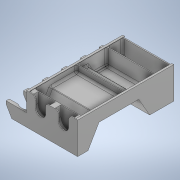
# Autodesk Inventor part: CardboardTray
Saved by Autodesk Inventor 2021 (Build 250183000, 183)
## iProperties
Created: 2023-03-18
Part Number: CardboardTray
Material: ABS Plastic
Document SubType Name: Modeling
Designer: Bradley
Density: 1.06 g/cm^3
Appearance: Smooth - Medium Gray
Author: Bradley
Autodesk Inventor part; units mm, degrees
ref_plane "YZ Plane" through (0, 0, 0) normal (1, 0, 0) x (0, 1, 0)
ref_plane "XZ Plane" through (0, 0, 0) normal (0, 1, 0) x (-1, 0, 0)
ref_plane "XY Plane" through (0, 0, 0) normal (0, 0, 1) x (1, 0, 0)
sketch "Sketch1" plane through (0, 0, 0) normal (1, 0, 0) x (0, 1, 0)
  line L0 (-22.4, 71.125) -> (-22.4, 55.7645)
  line L1 (-22.4, 55.7645) -> (5.9, 39.4255)
  line L2 (5.9, 39.4255) -> (5.9, -19.1755)
  line L3 (5.9, -19.1755) -> (-22.4, -35.5145)
  line L4 (-22.4, -35.5145) -> (-22.4, -71.125)
  line L5 (-22.4, -71.125) -> (22.4, -71.125)
  line L6 (22.4, -71.125) -> (22.4, 71.125)
  line L7 (22.4, 71.125) -> (-22.4, 71.125)
  line L8 (5.65, 39.2812) -> (5.65, -19.0312) construction
  line L9 (5.65, -19.0312) -> (-44.85, -48.1874) construction
  line L10 (-44.85, -48.1874) -> (-95.35, -19.0312) construction
  line L11 (-95.35, -19.0312) -> (-95.35, 39.2812) construction
  line L12 (-95.35, 39.2812) -> (-44.85, 68.4374) construction
  line L13 (-44.85, 68.4374) -> (5.65, 39.2812) construction
  line L14 (5.9, 39.4255) -> (5.9, -19.1755) construction
  line L15 (5.9, -19.1755) -> (-44.85, -48.4761) construction
  line L16 (-44.85, -48.4761) -> (-95.6, -19.1755) construction
  line L17 (-95.6, -19.1755) -> (-95.6, 39.4255) construction
  line L18 (-95.6, 39.4255) -> (-44.85, 68.7261) construction
  line L19 (-44.85, 68.7261) -> (5.9, 39.4255) construction
  line L20 (-22.4, -35.5145) -> (-22.4, 55.7645)
  point P0 (5.9, 10.125)
  point P1 (5.9, 10.125)
  point P2 (-44.85, 10.125)
  point P3 (0, 0)
  point P4 (22.4, 0)
  point P5 (0, 71.125)
  dimension "d0" = 101
  dimension "d1" = 61
  dimension "d2" = 0.25
  dimension "d3" = 73.2
  dimension "d4" = 142.25
  dimension "d5" = 44.8
  dimension "d80" = 16.5
  constraints: 42 end point, 3 collinear, 3 midpoint, 3 parallel, 3 perpendicular, 3 vertical, 2 point on line, 1 coincident, 1 horizontal alignment, 1 vertical alignment, 18 other
  measures "d0" distance between parallel lines of L11 L8
  measures "d1" distance from line of point (-44.85, 10.125) L7
  measures "d2" distance between parallel lines of L13 L19
  measures "d3" distance between parallel lines of L0 L17
  measures "d4" distance of L5.end L6.end
  measures "d5" distance of L6.end L0.start
  measures "d80" distance between parallel lines of L6 L2
extrude "Extrusion1" add sketch "Sketch1" along normal blind 64.6 contours L7 L6 L5 L4 L3 L2 L1 L0
extrude "Extrusion2" add sketch "Sketch1" against normal blind 11
sketch "Sketch2" plane through (64.6, -22.4, 71.125) normal (0, 0, 1) x (1, 0, 0)
  line L0 (-75.6, 0) -> (0, 0) projected
  line L1 (0, 44.8) -> (0, 0) projected
  line L2 (-75.6, 44.8) -> (0, 44.8) projected
  line L3 (-75.6, 0) -> (-75.6, 44.8) projected
  line L4 (-87.5152, -18) -> (-118.8076, -72.2) construction
  line L5 (-118.8076, -72.2) -> (-181.3924, -72.2) construction
  line L6 (-181.3924, -72.2) -> (-212.6848, -18) construction
  line L7 (-212.6848, -18) -> (-181.3924, 36.2) construction
  line L8 (-181.3924, 36.2) -> (-118.8076, 36.2) construction
  line L9 (-118.8076, 36.2) -> (-87.5152, -18) construction
  line L10 (-118.5189, 36.7) -> (-181.6811, 36.7) construction
  line L11 (-181.6811, 36.7) -> (-213.2621, -18) construction
  line L12 (-213.2621, -18) -> (-181.6811, -72.7) construction
  line L13 (-181.6811, -72.7) -> (-118.5189, -72.7) construction
  line L14 (-118.5189, -72.7) -> (-86.9379, -18) construction
  line L15 (-86.9379, -18) -> (-118.5189, 36.7) construction
  line L16 (-75.6, 0) -> (-97.3302, 0)
  line L17 (-97.3302, 0) -> (-105.6, 14.3237)
  line L18 (-105.6, 14.3237) -> (-105.6, 18.8)
  line L19 (-105.6, 18.8) -> (-75.6, 18.8)
  point P0 (-64.6, 22.4)
  point P1 (-150.1, -18)
  point P2 (-64.6, -73.2)
  point P3 (-64.6, -73.2)
  point P4 (-64.6, -73.2)
  dimension "d10" = 150.1
  dimension "d11" = 108.4
  dimension "d12" = 0.5
  dimension "d13" = 1
  dimension "d14" = 92
  dimension "d15" = 30
  dimension "d51" = 18.8
  dimension "d52" = 26
  constraints: 32 end point, 3 point on line, 2 horizontal, 1 perpendicular, 1 vertical, 18 other
  measures "d10" distance from line of point (-150.1, -18) L1
  measures "d11" distance between parallel lines of L5 L8
  measures "d12" distance between parallel lines of L8 L10
  measures "d13" distance from line of point (-64.6, -73.2) L5
  measures "d14" distance from line of point (-64.6, -73.2) L19
  measures "d15" distance between parallel lines of L18 L3
  measures "d51" distance between parallel lines of L16 L19
  measures "d52" distance between parallel lines of L2 L19
extrude "Extrusion3" add sketch "Sketch2" against normal up to surface (142.25 mm away) contours L16 L17 L18 L19 L3
sketch "Sketch6" plane through (-41, -3.6, 71.125) normal (0, 1, 0) x (1, 0, 0)
  circle A0 centre (21.0198, 15.0417) radius 12.75 construction
  circle A1 centre (21.0198, 15.0417) radius 13
  line L0 (30, 142.25) -> (0, 142.25) projected
  line L1 (0, 0) -> (0, 142.25) projected
  line L2 (30, 0) -> (0, 0) projected
  line L3 (30, 142.25) -> (30, 0) projected
  circle A2 centre (21.0198, 15.0417) radius 15.0417 construction
  line L4 (8.2698, 0) -> (105.6, 0) construction
  line L5 (8.2698, 0) -> (8.2698, 142.25) projected
  line L6 (0, 0) -> (0, 142.25) projected
  line L7 (0, 4.5417) -> (13.355, 4.5417)
  line L8 (13.355, 4.5417) -> (13.355, 25.5417)
  line L9 (13.355, 25.5417) -> (0, 25.5417)
  line L10 (0, 25.5417) -> (0, 4.5417)
  arc A3 (10.355, 4.5417) -> (10.355, 25.5417) centre (-6.52, 15.0417) ccw
  circle A4 centre (21.0198, 127.2083) radius 15.0417
  line L11 (21.0198, 15.0417) -> (21.0198, 127.2083) construction
  line L12 (30, 142.25) -> (0, 142.25) construction
  circle A5 centre (21.0198, 43.0833) radius 15.0417 construction
  point P0 (41, 71.125)
  point P1 (0, 25.5417)
  point P2 (30, 5.6419)
  point P3 (30, 24.4415)
  dimension "d43" = 25.5
  dimension "d44" = 2.0417
  dimension "d45" = 26
  dimension "d46" = 21
  dimension "d53" = 3
  dimension "d59" = 112.1667
  dimension "d60" = 30.0833
  dimension "d61" = 28.0417
  constraints: 10 end point, 6 centre point, 5 tangent, 4 point on circle, 4 point on line, 2 coincident, 2 equal radius, 2 parallel, 1 horizontal, 1 horizontal alignment, 1 perpendicular, 1 vertical
  measures "d43" diameter of A0
  measures "d44" radial gap between concentric circles of A1 A2
  measures "d45" diameter of A1
  measures "d46" distance of L7.end L8.end
  measures "d53" distance from line of A3.end L8
  measures "d59" distance of L11.start L11.end
  measures "d60" diameter of A2
  measures "d61" distance of A5.centre A0.centre
extrude "Extrusion5" cut sketch "Sketch6" along normal blind 26 and the other way blind 17.8 contours A1 L3 | L3 A1 L8 | L8 A3 A1 | A1 A3 L9 | L7 A3 A1 | A1 A3 L8 | A3 A1 L5 | A1 L5 L9 A3 | A3 L7 L5 A1 | L5 A1 | A1 L5 L7 L1 L9
extrude "Extrusion6" cut sketch "Sketch6" against normal through all contours A3 A1 L5 | A1 L5 L9 A3 | A3 L7 L5 A1 | L5 A1 | A1 L5 L7 L1 L9
pattern_linear "Rectangular Pattern2" count 5 spacing 28.0417 along (0, 0, -1) of "Extrusion5", "Extrusion6"
sketch "Sketch8" plane through (64.6, 22.4, 71.125) normal (0, 1, 0) x (1, 0, 0)
  line L0 (-67.7333, 9.2) -> (-41.7333, 9.2)
  line L1 (-41.7333, 9.2) -> (-41.7333, 1.2)
  line L2 (-41.7333, 1.2) -> (-67.7333, 1.2)
  line L3 (-67.7333, 1.2) -> (-67.7333, 9.2)
  line L4 (-33.8667, 9.2) -> (-7.8667, 9.2)
  line L5 (-7.8667, 9.2) -> (-7.8667, 1.2)
  line L6 (-7.8667, 1.2) -> (-33.8667, 1.2)
  line L7 (-33.8667, 1.2) -> (-33.8667, 9.2)
  arc A0 (-95.245, 4.5417) -> (-95.245, 25.5417) centre (-112.12, 15.0417) ccw projected
  line L8 (-92.245, 4.5417) -> (-95.245, 4.5417) projected
  arc A1 (-92.245, 4.5417) -> (-92.245, 25.5417) centre (-84.5802, 15.0417) ccw projected
  line L9 (-95.245, 25.5417) -> (-92.245, 25.5417) projected
  line L10 (-75.6, 0) -> (0, 0) projected
  line L11 (0, 142.25) -> (0, 0) projected
  point P0 (-64.6, 71.125)
  dimension "d67" = 13
  dimension "d68" = 26
  dimension "d69" = 1.2
  dimension "d70" = 7.8667
  dimension "d71" = 7.8667
  dimension "d72" = 7.8667
  dimension "d73" = 8
  constraints: 16 end point, 4 parallel, 2 horizontal, 2 perpendicular, 2 point on line, 1 collinear
  measures "d67" radius of A1
  measures "d68" distance of L0.start L0.end
  measures "d69" distance between parallel lines of L2 L10
  measures "d70" distance between parallel lines of L5 L11
  measures "d71" distance between parallel lines of L7 L1
  measures "d72" distance from line of L3 L10.start
  measures "d73" distance of L2.end L0.start
extrude "Extrusion8" cut sketch "Sketch8" against normal blind 27 contours L0 L1 L2 L3 | L4 L5 L6 L7
sketch "Sketch9" plane through (64.6, -22.4, 71.125) normal (0, 0, 1) x (1, 0, 0)
  line L0 (-67.7333, 44.8) -> (-41.7333, 44.8) projected
  line L1 (-67.7333, 44.8) -> (-67.7333, 17.8) projected
  line L2 (-67.7333, 17.8) -> (-41.7333, 17.8) projected
  line L3 (-41.7333, 44.8) -> (-41.7333, 17.8) projected
  line L4 (-33.8667, 44.8) -> (-7.8667, 44.8) projected
  line L5 (-33.8667, 44.8) -> (-33.8667, 17.8) projected
  line L6 (-33.8667, 17.8) -> (-7.8667, 17.8) projected
  line L7 (-7.8667, 44.8) -> (-7.8667, 17.8) projected
  line L8 (-75.6, 44.8) -> (0, 44.8) projected
  arc A0 (-62.2333, 40.8) -> (-66.2333, 44.8) centre (-66.2333, 40.8) ccw
  arc A1 (-43.2333, 44.8) -> (-47.2333, 40.8) centre (-43.2333, 40.8) ccw
  arc A2 (-62.2333, 30.8) -> (-47.2333, 30.8) centre (-54.7333, 30.8) ccw
  arc A3 (-28.3667, 40.8) -> (-32.3667, 44.8) centre (-32.3667, 40.8) ccw
  arc A4 (-9.3667, 44.8) -> (-13.3667, 40.8) centre (-9.3667, 40.8) ccw
  arc A5 (-28.3667, 30.8) -> (-13.3667, 30.8) centre (-20.8667, 30.8) ccw
  line L9 (-62.2333, 40.8) -> (-62.2333, 30.8)
  line L10 (-47.2333, 30.8) -> (-47.2333, 40.8)
  line L11 (-28.3667, 40.8) -> (-28.3667, 30.8)
  line L12 (-13.3667, 30.8) -> (-13.3667, 40.8)
  circle A6 centre (-54.7333, 30.8) radius 13 construction
  line L13 (-67.7333, 44.8) -> (-67.7333, 17.8) construction
  line L14 (-75.6, 44.8) -> (0, 44.8) construction
  point P0 (-64.6, 22.4)
  point P1 (-20.8667, 17.8)
  point P2 (-32.3667, 44.8)
  dimension "d76" = 4
  dimension "d77" = 15
  constraints: 12 point on circle, 11 tangent, 8 end point, 7 centre point, 4 equal radius, 4 parallel, 1 coincident, 1 midpoint, 1 point on line, 1 vertical, 1 vertical alignment, 9 other
  measures "d76" radius of A0
  measures "d77" distance between parallel lines of L10 L9
extrude "Extrusion9" cut sketch "Sketch9" against normal up to surface (1.2 mm away) contours L0 A1 L10 A2 L9 A0 | L4 A4 L12 A5 L11 A3
sketch "Sketch12" plane through (64.6, -22.4, 71.125) normal (0, 0, 1) x (1, 0, 0)
  line L0 (-71.5802, 1) -> (-71.5802, 44.8) projected
  arc A0 (-62.2333, 40.8) -> (-66.2333, 44.8) centre (-66.2333, 40.8) ccw projected
  line L1 (-75.6, 44.8) -> (-66.2333, 44.8) projected
  line L2 (-75.6, 18.8) -> (-75.6, 44.8) projected
  line L3 (-75.6, 18.8) -> (-105.6, 18.8) projected
  line L4 (-105.6, 18.8) -> (-105.6, 14.3237) projected
  line L5 (-105.6, 14.3237) -> (-97.3302, 0) projected
  line L6 (-97.3302, 0) -> (0, 0) projected
  line L7 (0, 44.8) -> (0, 0) projected
  line L8 (-9.3667, 44.8) -> (0, 44.8) projected
  arc A1 (-9.3667, 44.8) -> (-13.3667, 40.8) centre (-9.3667, 40.8) ccw projected
  line L9 (-13.3667, 40.8) -> (-13.3667, 30.8) projected
  arc A2 (-28.3667, 30.8) -> (-13.3667, 30.8) centre (-20.8667, 30.8) ccw projected
  line L10 (-28.3667, 30.8) -> (-28.3667, 40.8) projected
  arc A3 (-28.3667, 40.8) -> (-32.3667, 44.8) centre (-32.3667, 40.8) ccw projected
  line L11 (-43.2333, 44.8) -> (-32.3667, 44.8) projected
  arc A4 (-43.2333, 44.8) -> (-47.2333, 40.8) centre (-43.2333, 40.8) ccw projected
  line L12 (-47.2333, 40.8) -> (-47.2333, 30.8) projected
  arc A5 (-62.2333, 30.8) -> (-47.2333, 30.8) centre (-54.7333, 30.8) ccw projected
  line L13 (-62.2333, 30.8) -> (-62.2333, 40.8) projected
  line L14 (-71.5802, 1) -> (-71.5802, 44.8) projected
  line L15 (-71.5802, 18.8) -> (-75.6, 22.8198)
  line L16 (-75.6, 44.8) -> (-75.6, 18.8) projected
  line L17 (-75.6, 18.8) -> (-105.6, 18.8) projected
  point P0 (-64.6, 22.4)
  dimension "d96" = 135
  constraints: 3 point on line, 2 end point
  measures "d96" angle of L2 L15
extrude "Extrusion12" add sketch "Sketch12" against normal through all contours L15 L2 L1 L0
sketch "Sketch10" plane through (64.6, 22.4, 71.125) normal (0, 1, 0) x (1, 0, 0)
  line L0 (-66.2333, 1.2) -> (-66.2333, 0) projected
  line L1 (-66.2333, 1.2) -> (-67.7333, 1.2) projected
  line L2 (-67.7333, 1.2) -> (-67.7333, 9.2) projected
  line L3 (-67.7333, 9.2) -> (-41.7333, 9.2) projected
  line L4 (-41.7333, 9.2) -> (-41.7333, 1.2) projected
  line L5 (-41.7333, 1.2) -> (-43.2333, 1.2) projected
  line L6 (-43.2333, 1.2) -> (-43.2333, 0) projected
  line L7 (-43.2333, 0) -> (-32.3667, 0) projected
  line L8 (-32.3667, 1.2) -> (-32.3667, 0) projected
  line L9 (-32.3667, 1.2) -> (-33.8667, 1.2) projected
  line L10 (-33.8667, 1.2) -> (-33.8667, 9.2) projected
  line L11 (-33.8667, 9.2) -> (-7.8667, 9.2) projected
  line L12 (-7.8667, 9.2) -> (-7.8667, 1.2) projected
  line L13 (-7.8667, 1.2) -> (-9.3667, 1.2) projected
  line L14 (-9.3667, 1.2) -> (-9.3667, 0) projected
  line L15 (-9.3667, 0) -> (0, 0) projected
  line L16 (0, 142.25) -> (0, 0) projected
  line L17 (-75.6, 142.25) -> (0, 142.25) projected
  line L18 (-75.6, 0) -> (-75.6, 142.25) projected
  line L19 (-75.6, 0) -> (-66.2333, 0) projected
  line L20 (-67.7333, 1.2) -> (-67.7333, 9.2) projected
  circle A0 centre (-12.7327, 21.5327) radius 9.45 construction
  circle A1 centre (-12.7327, 21.5327) radius 11.1327 construction
  circle A2 centre (-32.7865, 21.5327) radius 11.1327 construction
  circle A3 centre (-52.8404, 21.5327) radius 11.1327 construction
  circle A4 centre (-22.7596, 41.4125) radius 11.1327 construction
  circle A5 centre (-42.8135, 41.4125) radius 11.1327 construction
  circle A6 centre (-62.8673, 41.4125) radius 11.1327 construction
  circle A7 centre (-12.7327, 61.2922) radius 11.1327 construction
  circle A8 centre (-12.7327, 129.5173) radius 11.1327 construction
  line L21 (-1.6, 10.4) -> (-74, 10.4)
  line L22 (-74, 10.4) -> (-74, 72.4249)
  line L23 (-74, 72.4249) -> (-1.6, 72.4249)
  line L24 (-1.6, 72.4249) -> (-1.6, 10.4)
  line L25 (-74, 73.6249) -> (-1.6, 73.6249)
  line L26 (-1.6, 73.6249) -> (-1.6, 117.1847)
  line L27 (-1.6, 117.1847) -> (-74, 117.1847)
  line L28 (-74, 117.1847) -> (-74, 73.6249)
  line L29 (-1.6, 118.3847) -> (-74, 118.3847)
  line L30 (-74, 118.3847) -> (-74, 140.65)
  line L31 (-74, 140.65) -> (-1.6, 140.65)
  line L32 (-1.6, 140.65) -> (-1.6, 118.3847)
  line L33 (-64.6, 90.3005) -> (0, 90.3005) projected
  line L34 (-64.6, 106.6395) -> (0, 106.6395) projected
  line L35 (0, 142.25) -> (0, 0) construction
  line L36 (0, 94.9193) -> (-64.6, 94.9193) construction
  line L37 (0, 90.3005) -> (8, 94.9193) construction
  circle A9 centre (-12.7327, 106.052) radius 11.1327 construction
  dimension "d82" = 18.9
  dimension "d83" = 22.2653
  dimension "d99" = 1.2
  dimension "d100" = 1.6
  dimension "d101" = 1.6
  dimension "d102" = 1.6
  dimension "d103" = 1.2
  dimension "d104" = 1.2
  dimension "d105" = 22.2653
  dimension "d106" = 62.0249
  dimension "d133" = 120
  dimension "d134" = 8
  constraints: 28 end point, 19 tangent, 10 centre point, 8 equal radius, 6 parallel, 4 collinear, 4 horizontal, 3 perpendicular, 2 horizontal alignment, 2 point on line, 1 coincident, 1 vertical alignment
  measures "d82" diameter of A0
  measures "d83" diameter of A1
  measures "d99" distance between parallel lines of L21 L3
  measures "d100" distance between parallel lines of L18 L22
  measures "d101" distance between parallel lines of L17 L31
  measures "d102" distance between parallel lines of L16 L24
  measures "d103" distance between parallel lines of L23 L25
  measures "d104" distance between parallel lines of L29 L27
  measures "d105" distance of L31.end L29.start
  measures "d106" distance of L23.end L21.start
  measures "d133" angle of L16 L37
  measures "d134" horizontal distance of L33.end L37.end
ref_plane "Work Plane1" through (63, 22.4, -69.525) normal (0, 0, -1) x (-1, 0, 0)
sketch "Sketch13" plane through (63, 22.4, -69.525) normal (0, 0, -1) x (-1, 0, 0)
  line L0 (74, 0) -> (-1.6, 0) projected
  line L1 (-1.6, -44.8) -> (-1.6, 0) projected
  line L2 (95.7302, -44.8) -> (-1.6, -44.8) projected
  line L3 (104, -30.4763) -> (95.7302, -44.8) projected
  line L4 (104, -26) -> (104, -30.4763) projected
  line L5 (74, -26) -> (104, -26) projected
  line L6 (74, 0) -> (74, -26) projected
  line L7 (74, -21.9802) -> (69.9802, -26) projected
  line L8 (74, -21.9802) -> (74, -21.9802) projected
  line L9 (74, -26) -> (74, -21.9802) projected
  line L10 (90.645, -26) -> (74, -26) projected
  line L11 (90.645, -43.8) -> (90.645, -26) projected
  line L12 (90.645, -43.8) -> (90.645, -43.8) projected
  line L13 (90.645, -43.8) -> (90.645, -26) projected
  line L14 (74, -26) -> (90.645, -26) projected
  line L15 (74, -21.9802) -> (74, -26) projected
  line L16 (0, -43.8) -> (68.3802, -43.8)
  line L17 (68.3802, -43.8) -> (68.3802, -25.9029)
  line L18 (68.3802, -25.9029) -> (72.4, -21.8831)
  line L19 (72.4, -21.8831) -> (72.4, 0)
  line L20 (0, -43.8) -> (0, 0)
  point P0 (63, -22.4)
  point P1 (0, 0)
  point P2 (72.4, 0)
  point P3 (72.4, 0)
  dimension "d107" = 1
  dimension "d108" = 1.2
  dimension "d109" = 1.6
  constraints: 10 end point, 3 parallel, 1 horizontal, 1 perpendicular
  measures "d107" distance between parallel lines of L2 L16
  measures "d108" distance between parallel lines of L18 L7
  measures "d109" distance from line of L7.end L17
extrude "Extrusion13" cut sketch "Sketch13" against normal up to surface (22.2653 mm away) contours L19 L18 L17 L16 L20 L0
extrude "Extrusion11" cut sketch "Sketch10" against normal blind 10 contours L26 L25 L28 L27 | L21 L22 L23 L24
sketch "Sketch14" plane through (63, 22.4, -46.0597) normal (-1, 0, 0) x (0, 0, 1)
  line L0 (0, 0) -> (43.5598, 0) projected
  line L1 (0, 0) -> (0, -10) projected
  line L2 (0, -10) -> (43.5598, -10) projected
  line L3 (43.5598, 0) -> (43.5598, -10) projected
  line L4 (44.7598, 0) -> (106.7847, 0) projected
  line L5 (44.7598, 0) -> (44.7598, -10) projected
  line L6 (44.7598, -10) -> (106.7847, -10) projected
  line L7 (106.7847, 0) -> (106.7847, -10) projected
  line L8 (101.8242, -44.8) -> (85.4852, -16.5) projected
  line L9 (85.4852, -16.5) -> (26.8841, -16.5) projected
  line L10 (26.8841, -16.5) -> (10.5451, -44.8) projected
  line L11 (10.5451, -44.8) -> (-25.0653, -44.8) projected
  line L12 (-25.0653, -44.8) -> (-25.0653, 0) projected
  line L13 (-25.0653, 0) -> (117.1847, 0) projected
  line L14 (117.1847, 0) -> (117.1847, -44.8) projected
  line L15 (117.1847, -44.8) -> (101.8242, -44.8) projected
  line L16 (44.7598, -10) -> (106.7847, -10) projected
  line L17 (106.7847, -10) -> (106.7847, -24)
  line L18 (106.7847, -24) -> (91.201, -24)
  line L19 (91.201, -24) -> (83.1181, -10)
  line L20 (0, -10) -> (0, -24)
  line L21 (0, -24) -> (21.1684, -24)
  line L22 (0, -10) -> (43.5598, -10) projected
  line L23 (29.2513, -10) -> (21.1684, -24)
  line L24 (-23.4653, -21.8831) -> (-1.2, -21.8831) projected
  line L25 (0, -21.8831) -> (22.3905, -21.8831)
  line L26 (106.7847, -21.8831) -> (89.9788, -21.8831)
  point P0 (46.0597, -22.4)
  point P1 (83.1181, -10)
  dimension "d112" = 15.5837
  dimension "d113" = 1.2
  dimension "d114" = 24
  dimension "d115" = 1.2
  dimension "d116" = 21.1684
  constraints: 16 end point, 6 point on line, 4 collinear, 2 parallel, 2 perpendicular, 2 vertical, 1 horizontal
  measures "d112" distance of L17.end L18.end
  measures "d113" distance between parallel lines of L19 L8
  measures "d114" distance between parallel lines of L18 L4
  measures "d115" distance between parallel lines of L10 L23
  measures "d116" distance of L20.end L21.end
extrude "Extrusion14" cut sketch "Sketch14" along normal up to surface (72.4 mm away) contours L2 L23 L25 L20 | L17 L26 L19 L6
extrude "Extrusion15" cut sketch "Sketch14" along normal up to surface contours L25 L23 L21 L20 | L17 L18 L19 L26 surface through (-9.4, 0.5169, -69.525) normal (-0.7071068, -0.7071068, 0)
fillet "Fillet2" radius 3 45 edges at (63, 0.5, -69.525) (63, 0.5, -47.2597) (63, -21.4, -58.3923) (28.8099, -21.4, -47.2597) (28.8099, -21.4, -69.525) (-5.3802, -21.4, -58.3923) (-5.3802, -12.4515, -69.525) (-7.3901, -1.493, -69.525) (-9.4, 11.4584, -69.525) (-9.4, 0.5169, -58.3923) (-5.3802, -3.5029, -58.3923) (-5.3802, -12.4515, -47.2597) (-7.3901, -1.493, -47.2597) (-9.4, 11.4584, -47.2597) (63, 10.4, -46.0597) (63, -1.6, -35.4755) (27.8584, -1.6, -46.0597) (63, 5.4, -20.8498) (63, 12.4, -9.6541) (27.8584, -1.6, -24.8913) (63, 17.4, -2.4999) (63, 17.4, -1.2999) (26.8, 12.4, -1.2999) (26.8, 12.4, -2.4999) (63, 12.4, 17.8792) (-9.4, 12.4, -9.6541) (-9.4, 6.4584, -20.2388) (-9.4, 0.5169, -34.8644) (-7.2831, -1.6, -35.4755) (-8.3416, -0.5416, -46.0597) (-9.4, 11.4584, -46.0597) (-8.3416, -0.5416, -24.2802) (-9.4, 12.4, 17.8792) (-9.4, 6.4584, 40.4888) (-9.4, 0.5169, 52.3221) (-8.3416, -0.5416, 44.5302) (-7.2831, -1.6, 52.9331) (27.8584, -1.6, 45.1413) (-9.4, 17.4, -1.2999) (-9.4, 11.4584, 60.725) (-8.3416, -0.5416, 60.725) (63, 10.4, 60.725) (63, -1.6, 52.9331) (27.8584, -1.6, 60.725) (63, 5.4, 41.0998)
fillet "Fillet2" radius 1 2 edges at (26.8, 12.4, 37.0584) (26.8, 12.4, -16.8084)
fillet "Fillet2" radius 12 4 edges at (-3.1333, -4.6, 65.925) (30.7333, -4.6, 65.925) (22.8667, -4.6, 65.925) (56.7333, -4.6, 65.925)
sketch "Sketch15" plane through (64.6, -22.4, -71.125) normal (0, 0, -1) x (-1, 0, 0)
  line L0 (75.6, 44.8) -> (0, 44.8) projected
  line L1 (0, 0) -> (0, 44.8) projected
  line L2 (97.3302, 0) -> (0, 0) projected
  line L3 (105.6, 14.3237) -> (97.3302, 0) projected
  line L4 (105.6, 18.8) -> (105.6, 14.3237) projected
  line L5 (75.6, 18.8) -> (105.6, 18.8) projected
  line L6 (75.6, 44.8) -> (75.6, 18.8) projected
  line L7 (75.6, 44.8) -> (0, 44.8) projected
  line L8 (0, 44.8) -> (0, 46.8)
  line L9 (0, 46.8) -> (3.1, 46.8)
  line L10 (4.6, 44.8) -> (1.6, 44.8) projected
  line L11 (3.1, 46.8) -> (1.6, 44.8)
  line L12 (75.6, 44.8) -> (75.6, 18.8) projected
  line L13 (75.6, 44.8) -> (75.6, 46.8)
  line L14 (75.6, 46.8) -> (72.5, 46.8)
  line L15 (4.6, 44.8) -> (74, 44.8) projected
  line L16 (72.5, 46.8) -> (74, 44.8)
  point P0 (64.6, 22.4)
  dimension "d124" = 2
  dimension "d125" = 1.5
  dimension "d126" = 53.13
  constraints: 12 end point, 2 collinear, 2 perpendicular, 2 vertical
  measures "d124" distance of L0.end L8.end
  measures "d125" horizontal distance of L10.end L9.end
  measures "d126" angle of L11 L9
extrude "Extrusion16" add sketch "Sketch15" against normal up to surface (142.25 mm away) contours L0 L16 L14 L13 | L0 L8 L9 L11
sketch "Sketch16" plane through (-41, -3.6, 71.125) normal (0, 0, 1) x (1, 0, 0)
  line L0 (30, 0) -> (30, 28) projected
  line L1 (30, 0) -> (0, 0) projected
  line L2 (0, 0) -> (0, -4.4763) projected
  line L3 (0, -4.4763) -> (8.2698, -18.8) projected
  line L4 (8.2698, -18.8) -> (105.6, -18.8) projected
  line L5 (105.6, 28) -> (105.6, -18.8) projected
  line L6 (102.5, 28) -> (105.6, 28) projected
  line L7 (104, 26) -> (102.5, 28) projected
  line L8 (96.2333, 26) -> (104, 26) projected
  arc A0 (96.2333, 26) -> (92.2333, 22) centre (96.2333, 22) ccw projected
  line L9 (92.2333, 22) -> (92.2333, 12) projected
  arc A1 (77.2333, 12) -> (92.2333, 12) centre (84.7333, 12) ccw projected
  line L10 (77.2333, 12) -> (77.2333, 22) projected
  arc A2 (77.2333, 22) -> (73.2333, 26) centre (73.2333, 22) ccw projected
  line L11 (62.3667, 26) -> (73.2333, 26) projected
  arc A3 (62.3667, 26) -> (58.3667, 22) centre (62.3667, 22) ccw projected
  line L12 (58.3667, 22) -> (58.3667, 12) projected
  arc A4 (43.3667, 12) -> (58.3667, 12) centre (50.8667, 12) ccw projected
  line L13 (43.3667, 12) -> (43.3667, 22) projected
  arc A5 (43.3667, 22) -> (39.3667, 26) centre (39.3667, 22) ccw projected
  line L14 (31.6, 26) -> (39.3667, 26) projected
  line L15 (33.1, 28) -> (31.6, 26) projected
  line L16 (30, 28) -> (33.1, 28) projected
  line L17 (33.1, 28) -> (31.6, 26) projected
  line L18 (33.1, 28) -> (40, 28)
  line L19 (31.6, 26) -> (39.3667, 26) projected
  line L20 (40, 28) -> (42.623, 24.3229)
  arc A6 (43.3667, 22) -> (39.3667, 26) centre (39.3667, 22) ccw projected
  line L21 (104, 26) -> (102.5, 28) projected
  line L22 (102.5, 28) -> (95.6, 28)
  line L23 (95.6, 28) -> (92.977, 24.3229)
  arc A7 (96.2333, 26) -> (92.2333, 22) centre (96.2333, 22) ccw projected
  point P0 (41, 3.6)
  dimension "d129" = 10
  dimension "d130" = 10
  constraints: 8 end point, 2 point on circle, 2 tangent, 1 parallel, 1 point on line
  measures "d129" distance from line of L22.end L5
  measures "d130" distance from line of L18.end L0
extrude "Extrusion17" add sketch "Sketch16" against normal up to surface (1.2 mm away) contours L18 L20 A5 L14 L15 | L7 L8 A0 L23 L22
sketch "Sketch17" plane through (-3.1333, 22.4, 61.925) normal (0, 1, 0) x (1, 0, 0)
  line L0 (26, -8) -> (24.5, -8) projected
  line L1 (0, -8) -> (0, 0) projected
  line L2 (0, 0) -> (26, 0) projected
  line L3 (26, 0) -> (26, -8) projected
  line L4 (24.5, -8) -> (24.5, -9.2) projected
  line L5 (24.5, -9.2) -> (35.3667, -9.2) projected
  line L6 (35.3667, -8) -> (35.3667, -9.2) projected
  line L7 (35.3667, -8) -> (33.8667, -8) projected
  line L8 (33.8667, -8) -> (33.8667, 0) projected
  line L9 (33.8667, 0) -> (59.8667, 0) projected
  line L10 (59.8667, 0) -> (59.8667, -8) projected
  line L11 (66.1333, 128.45) -> (66.1333, 133.05) projected
  arc A0 (63.1333, 1.2) -> (66.1333, 4.2) centre (63.1333, 4.2) ccw projected
  line L12 (63.1333, 1.2) -> (-3.2667, 1.2) projected
  arc A1 (-6.2667, 4.2) -> (-3.2667, 1.2) centre (-3.2667, 4.2) ccw projected
  line L13 (-6.2667, 4.2) -> (-6.2667, -8) projected
  line L14 (66.1333, -6.25) -> (65.7833, -6.0479)
  line L15 (65.5333, -5.6149) -> (65.5333, -4.3851)
  line L16 (65.7833, -3.9521) -> (66.1333, -3.75)
  arc A2 (65.7833, -3.9521) -> (65.5333, -4.3851) centre (66.0333, -4.3851) ccw
  arc A3 (65.5333, -5.6149) -> (65.7833, -6.0479) centre (66.0333, -5.6149) ccw
  line L17 (-6.2667, -6.25) -> (-5.9167, -6.0479)
  arc A4 (-5.9167, -6.0479) -> (-5.6667, -5.6149) centre (-6.1667, -5.6149) ccw
  line L18 (-5.6667, -5.6149) -> (-5.6667, -4.3851)
  arc A5 (-5.6667, -4.3851) -> (-5.9167, -3.9521) centre (-6.1667, -4.3851) ccw
  line L19 (-5.9167, -3.9521) -> (-6.2667, -3.75)
  line L20 (-6.2667, 64.4249) -> (-6.2667, 60.2249) projected
  arc A6 (-3.2667, 63.2249) -> (-6.2667, 60.2249) centre (-3.2667, 60.2249) ccw projected
  line L21 (-3.2667, 63.2249) -> (63.1333, 63.2249) projected
  arc A7 (66.1333, 60.2249) -> (63.1333, 63.2249) centre (63.1333, 60.2249) ccw projected
  line L22 (66.1333, 60.2249) -> (66.1333, 67.4249) projected
  arc A8 (63.1333, 64.4249) -> (66.1333, 67.4249) centre (63.1333, 67.4249) ccw projected
  line L23 (63.1333, 64.4249) -> (-6.2667, 64.4249) projected
  line L24 (-6.2667, 112.1847) -> (-6.2667, 104.9847) projected
  arc A9 (-3.2667, 107.9847) -> (-6.2667, 104.9847) centre (-3.2667, 104.9847) ccw projected
  line L25 (-3.2667, 107.9847) -> (63.1333, 107.9847) projected
  arc A10 (66.1333, 104.9847) -> (63.1333, 107.9847) centre (63.1333, 104.9847) ccw projected
  line L26 (66.1333, 104.9847) -> (66.1333, 112.1847) projected
  arc A11 (63.1333, 109.1847) -> (66.1333, 112.1847) centre (63.1333, 112.1847) ccw projected
  line L27 (63.1333, 109.1847) -> (-3.2667, 109.1847) projected
  arc A12 (-6.2667, 112.1847) -> (-3.2667, 109.1847) centre (-3.2667, 112.1847) ccw projected
  line L28 (-6.2667, 133.05) -> (-6.2667, 128.45) projected
  arc A13 (-3.2667, 131.45) -> (-6.2667, 128.45) centre (-3.2667, 128.45) ccw projected
  line L29 (-3.2667, 131.45) -> (63.1333, 131.45) projected
  arc A14 (66.1333, 128.45) -> (63.1333, 131.45) centre (63.1333, 128.45) ccw projected
  line L30 (-6.2667, 133.05) -> (66.1333, 133.05) projected
  line L31 (-6.2667, -8) -> (0, -8) projected
  line L32 (59.8667, -8) -> (66.1333, -8) projected
  line L33 (66.1333, -8) -> (66.1333, 4.2) projected
  point P0 (3.1333, 61.925)
  point P1 (65.5333, -5)
  point P2 (-5.6667, -5)
  point P3 (66.1333, -6.25)
  point P4 (66.1333, -3.75)
  dimension "d135" = 0.5
  dimension "d136" = 0.6
  dimension "d137" = 60
  dimension "d139" = 2.5
  dimension "d143" = 3
  constraints: 12 end point, 8 point on circle, 8 tangent, 4 centre point, 4 equal length, 4 point on line, 3 equal radius, 2 horizontal alignment, 2 midpoint, 2 vertical
  measures "d135" radius of A2
  measures "d136" distance between parallel lines of L15 L11
  measures "d137" angle of L16 L14
  measures "d139" distance of L16.end L14.start
  measures "d143" distance from line of point (65.533, -5) L32
extrude "Extrusion18" add sketch "Sketch17" along normal up to surface (2 mm away) contours L13 L19 A5 L18 A4 L17 | L14 A3 L15 A2 L16 L33
equation "\"d61\" = 0.25 * d59"
equation "\"d47\" = d52"
equation "\"d58\" = 0.25 * d59"
equation "\"d68\" = 2 * d67"
equation "\"d70\" = d72"
equation "\"d71\" = d70"
equation "\"d78\" = d68"
equation "\"d102\" = d100"
equation "\"d103\" = d99"
equation "\"d104\" = d103"
equation "\"d109\" = d100"
equation "\"d115\" = d113"
body "Solid1"
